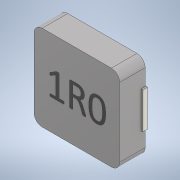
# Autodesk Inventor part: L_52x54x18mm
Saved by Autodesk Inventor 2020 (Build 240168000, 168)
## iProperties
Created: 2020-07-25
Part Number: L_52x54x18mm
Material: Generic
Document SubType Name: Modeling
Designer: franc
Density: 1 g/cm^3
Appearance: Default
Author: franc
Autodesk Inventor part; units mm, degrees
ref_plane "YZ Plane" through (0, 0, 0) normal (1, 0, 0) x (0, 1, 0)
ref_plane "XZ Plane" through (0, 0, 0) normal (0, 1, 0) x (-1, 0, 0)
ref_plane "XY Plane" through (0, 0, 0) normal (0, 0, 1) x (1, 0, 0)
sketch "Sketch1" plane through (0, 0, 0) normal (0, 0, 1) x (1, 0, 0)
  line L0 (-2.6, 2.6) -> (2.6, 2.6)
  line L1 (2.6, 2.6) -> (2.6, -2.6)
  line L2 (2.6, -2.6) -> (-2.6, -2.6)
  line L3 (-2.6, -2.6) -> (-2.6, 2.6)
  line L4 (-2.6, 2.6) -> (2.6, -2.6) construction
  line L5 (2.6, 2.6) -> (-2.6, -2.6) construction
  point P0 (0, 0)
  dimension "d0" = 5.2
  dimension "d1" = 5.2
  constraints: 12 end point, 2 midpoint, 2 parallel, 1 horizontal, 1 perpendicular
  measures "d0" distance of L0.start L0.end
  measures "d1" distance of L0.end L1.end
extrude "Extrusion1" add sketch "Sketch1" along normal blind 1.55
sketch "Sketch2" plane through (0, 0, 0) normal (0, 0, -1) x (-1, 0, 0)
  line L0 (-1.5, -1.1) -> (-2.7, -1.1)
  line L1 (-2.7, -1.1) -> (-2.7, 1.1)
  line L2 (-2.7, 1.1) -> (-1.5, 1.1)
  line L3 (-1.5, 1.1) -> (-1.5, -1.1)
  line L4 (-1.5, -1.1) -> (-2.7, 1.1) construction
  line L5 (-2.7, -1.1) -> (-1.5, 1.1) construction
  line L6 (-2.6, -2.6) -> (-2.6, 2.6) construction
  line L7 (-2.6, 0) -> (2.6, 0) construction
  line L8 (2.6, 2.6) -> (2.6, -2.6) construction
  line L9 (-2.6, 2.6) -> (2.6, 2.6) construction
  line L10 (0, 2.6) -> (0, 0) construction
  line L11 (1.5, -1.1) -> (2.7, -1.1)
  line L12 (2.7, -1.1) -> (2.7, 1.1)
  line L13 (2.7, 1.1) -> (1.5, 1.1)
  line L14 (1.5, 1.1) -> (1.5, -1.1)
  point P0 (-2.1, 0)
  point P1 (-2.1, 0)
  point P2 (2.1, 0)
  point P3 (2.1, 0)
  dimension "d4" = 1.2
  dimension "d5" = 0.1
  dimension "d6" = 2.2
  dimension "d7" = 5.4
  constraints: 24 end point, 6 midpoint, 6 symmetric about line, 2 parallel, 1 horizontal, 1 perpendicular, 1 point on line, 1 vertical
  measures "d4" distance of L0.start L0.end
  measures "d5" distance between parallel lines of L6 L1
  measures "d6" distance of L0.end L1.end
  measures "d7" distance between parallel lines of L12 L1
extrude "Extrusion2" add sketch "Sketch2" along normal blind 0.05 and the other way blind 0.25
fillet "Fillet1" radius 0.5 4 edges at (2.6, 2.6, 0.775) (-2.6, 2.6, 0.775) (2.6, -2.6, 0.775) (-2.6, -2.6, 0.775)
sketch "Sketch3" plane through (0, 0, 1.55) normal (0, 0, 1) x (1, 0, 0)
  line L0 (-2.5, 1.25) -> (2.5, 1.25) construction
  line L1 (2.5, 1.25) -> (2.5, -1.25) construction
  line L2 (2.5, -1.25) -> (-2.5, -1.25) construction
  line L3 (-2.5, -1.25) -> (-2.5, 1.25) construction
  line L4 (2.1, 2.6) -> (-2.1, 2.6) construction
  line L5 (0, 2.6) -> (0, -2.6) construction
  line L6 (-2.1, -2.6) -> (2.1, -2.6) construction
  line L7 (-2.6, 1.1) -> (-2.6, -1.1) construction
  line L8 (-2.6, 0) -> (2.6, 0) construction
  line L9 (2.6, -1.1) -> (2.6, 1.1) construction
  spline S0 degree 2 poles (-0.7697, -0.6676) (-0.7697, -0.6901) (-0.7768, -0.7197) (-0.788, -0.738) (-0.8035, -0.7465) (-0.8106, -0.7465) knots 0 0 0 1 2 3 4 4 4
  line L10 (-0.8106, -0.7465) -> (-1.5908, -0.7465)
  spline S1 degree 2 poles (-1.5908, -0.7465) (-1.5993, -0.7465) (-1.6134, -0.738) (-1.6261, -0.7197) (-1.6331, -0.6901) (-1.6331, -0.6676) knots 0 0 0 1 2 3 4 4 4
  spline S2 degree 2 poles (-1.6331, -0.6676) (-1.6331, -0.6479) (-1.6261, -0.6169) (-1.6162, -0.5972) (-1.6007, -0.5873) (-1.5908, -0.5873) knots 0 0 0 1 2 3 4 4 4
  line L11 (-1.5908, -0.5873) -> (-1.2796, -0.5873)
  line L12 (-1.2796, -0.5873) -> (-1.2796, 0.5493)
  line L13 (-1.2796, 0.5493) -> (-1.5683, 0.3775)
  spline S3 degree 2 poles (-1.5683, 0.3775) (-1.5908, 0.3662) (-1.6162, 0.362) (-1.6331, 0.3761) (-1.6387, 0.4113) (-1.6387, 0.438) knots 0 0 0 1 2 3 4 4 4
  spline S4 degree 2 poles (-1.6387, 0.438) (-1.6387, 0.4563) (-1.6359, 0.4845) (-1.6289, 0.5028) (-1.6162, 0.5169) (-1.6049, 0.5239) knots 0 0 0 1 2 3 4 4 4
  line L14 (-1.6049, 0.5239) -> (-1.2613, 0.7437)
  spline S5 degree 2 poles (-1.2613, 0.7437) (-1.257, 0.7479) (-1.243, 0.7521) (-1.2218, 0.7563) (-1.1937, 0.7577) (-1.1739, 0.7577) knots 0 0 0 1 2 3 4 4 4
  spline S6 degree 2 poles (-1.1739, 0.7577) (-1.1458, 0.7577) (-1.1092, 0.7535) (-1.088, 0.7451) (-1.081, 0.7324) (-1.081, 0.7254) knots 0 0 0 1 2 3 4 4 4
  line L15 (-1.081, 0.7254) -> (-1.081, -0.5873)
  line L16 (-1.081, -0.5873) -> (-0.8106, -0.5873)
  spline S7 degree 2 poles (-0.8106, -0.5873) (-0.8021, -0.5873) (-0.7852, -0.5972) (-0.7754, -0.6169) (-0.7697, -0.6479) (-0.7697, -0.6676) knots 0 0 0 1 2 3 4 4 4
  spline S8 degree 2 poles (0.5528, -0.7169) (0.5528, -0.7254) (0.5458, -0.7394) (0.5232, -0.7493) (0.481, -0.7535) (0.4472, -0.7535) knots 0 0 0 1 2 3 4 4 4
  spline S9 degree 2 poles (0.4472, -0.7535) (0.4162, -0.7535) (0.3782, -0.7493) (0.3556, -0.738) (0.343, -0.7197) (0.3387, -0.7056) knots 0 0 0 1 2 3 4 4 4
  line L17 (0.3387, -0.7056) -> (0.2007, -0.3549)
  spline S10 degree 2 poles (0.2007, -0.3549) (0.1768, -0.2944) (0.1246, -0.1944) (0.0528, -0.1225) (-0.043, -0.0817) (-0.112, -0.0817) knots 0 0 0 1 2 3 4 4 4
  line L18 (-0.112, -0.0817) -> (-0.2444, -0.0817)
  line L19 (-0.2444, -0.0817) -> (-0.2444, -0.7169)
  spline S11 degree 2 poles (-0.2444, -0.7169) (-0.2444, -0.7254) (-0.2542, -0.7394) (-0.2768, -0.7479) (-0.3148, -0.7535) (-0.343, -0.7535) knots 0 0 0 1 2 3 4 4 4
  spline S12 degree 2 poles (-0.343, -0.7535) (-0.3725, -0.7535) (-0.4106, -0.7479) (-0.4331, -0.7394) (-0.443, -0.7254) (-0.443, -0.7169) knots 0 0 0 1 2 3 4 4 4
  line L20 (-0.443, -0.7169) -> (-0.443, 0.6662)
  spline S13 degree 2 poles (-0.443, 0.6662) (-0.443, 0.7113) (-0.3951, 0.7465) (-0.3697, 0.7465) knots 0 0 0 1 2 2 2
  line L21 (-0.3697, 0.7465) -> (-0.0514, 0.7465)
  spline S14 degree 2 poles (-0.0514, 0.7465) (0.0049, 0.7465) (0.0796, 0.7408) (0.1092, 0.7366) knots 0 0 0 1 2 2 2
  spline S15 degree 2 poles (0.1092, 0.7366) (0.1965, 0.7225) (0.3289, 0.6577) (0.419, 0.5577) (0.4641, 0.4296) (0.4641, 0.3521) knots 0 0 0 1 2 3 4 4 4
  spline S16 degree 2 poles (0.4641, 0.3521) (0.4641, 0.2775) (0.4232, 0.1592) (0.3472, 0.0676) (0.2415, 0) (0.1754, -0.0225) knots 0 0 0 1 2 3 4 4 4
  spline S17 degree 2 poles (0.1754, -0.0225) (0.212, -0.0394) (0.2725, -0.0887) (0.3246, -0.1577) (0.3711, -0.2479) (0.3937, -0.3042) knots 0 0 0 1 2 3 4 4 4
  line L22 (0.3937, -0.3042) -> (0.5275, -0.6324)
  spline S18 degree 2 poles (0.5275, -0.6324) (0.5444, -0.6746) (0.5528, -0.707) (0.5528, -0.7169) knots 0 0 0 1 2 2 2
  spline S19 degree 2 poles (0.2542, 0.3324) (0.2542, 0.4197) (0.1754, 0.5408) (0.0838, 0.5676) knots 0 0 0 1 2 2 2
  spline S20 degree 2 poles (0.0838, 0.5676) (0.0542, 0.5761) (-0.0176, 0.5831) (-0.0768, 0.5831) knots 0 0 0 1 2 2 2
  line L23 (-0.0768, 0.5831) -> (-0.2444, 0.5831)
  line L24 (-0.2444, 0.5831) -> (-0.2444, 0.0789)
  line L25 (-0.2444, 0.0789) -> (-0.05, 0.0789)
  spline S21 degree 2 poles (-0.05, 0.0789) (0.0275, 0.0789) (0.143, 0.1169) (0.219, 0.1859) (0.2542, 0.2775) (0.2542, 0.3324) knots 0 0 0 1 2 3 4 4 4
  spline S22 degree 2 poles (1.757, 0.0028) (1.757, -0.169) (1.7035, -0.4521) (1.5768, -0.6563) (1.3739, -0.769) (1.2246, -0.769) knots 0 0 0 1 2 3 4 4 4
  spline S23 degree 2 poles (1.2246, -0.769) (1.0852, -0.769) (0.8923, -0.669) (0.7739, -0.4732) (0.7246, -0.1887) (0.7246, -0.0028) knots 0 0 0 1 2 3 4 4 4
  spline S24 degree 2 poles (0.7246, -0.0028) (0.7246, 0.1676) (0.7796, 0.4521) (0.9049, 0.6563) (1.1077, 0.769) (1.2556, 0.769) knots 0 0 0 1 2 3 4 4 4
  spline S25 degree 2 poles (1.2556, 0.769) (1.3965, 0.769) (1.5894, 0.669) (1.7077, 0.4732) (1.757, 0.1887) (1.757, 0.0028) knots 0 0 0 1 2 3 4 4 4
  spline S26 degree 2 poles (1.5542, -0.0099) (1.5542, 0.1014) (1.5387, 0.2789) (1.5063, 0.4155) (1.457, 0.5127) (1.388, 0.5775) (1.2993, 0.6056) (1.2444, 0.6056) knots 0 0 0 1 2 3 4 5 6 6 6
  spline S27 degree 2 poles (1.2444, 0.6056) (1.1458, 0.6056) (1.0232, 0.5127) (0.9528, 0.3521) (0.9275, 0.1352) (0.9275, 0.0099) knots 0 0 0 1 2 3 4 4 4
  spline S28 degree 2 poles (0.9275, 0.0099) (0.9275, -0.1563) (0.9627, -0.3915) (1.0373, -0.538) (1.1542, -0.6056) (1.2373, -0.6056) knots 0 0 0 1 2 3 4 4 4
  spline S29 degree 2 poles (1.2373, -0.6056) (1.3021, -0.6056) (1.3993, -0.5648) (1.4697, -0.4873) (1.5162, -0.3789) (1.5444, -0.2465) (1.5542, -0.093) (1.5542, -0.0099) knots 0 0 0 1 2 3 4 5 6 6 6
  point P0 (0, 0)
  dimension "d13" = 5
  dimension "d14" = 2.5
  constraints: 4 end point, 4 midpoint, 1 symmetric about line, 3 other
  measures "d13" distance of L2.end L1.end
  measures "d14" distance of L1.end L0.end
extrude "Extrusion4" cut sketch "Sketch3" against normal blind 0.01
body "Solid1"
